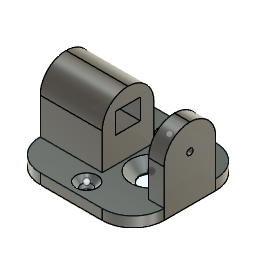
motorframe (Autodesk Fusion 360 design; units mm, degrees)
Autodesk Fusion 360 part; units mm, degrees
sketch "Skizze3" plane through (0, 0, 0) normal (0, 0, 1) x (1, 0, 0)
  line L0 (0, 0) -> (60, 0)
  line L1 (60, 0) -> (60, 55)
  line L2 (60, 55) -> (0, 55)
  line L3 (0, 55) -> (0, 0)
  line L4 (60, 55) -> (0, 55)
  line L5 (0, 55) -> (0, 0)
  line L6 (0, 0) -> (60, 0)
  line L7 (60, 0) -> (60, 55)
  line L8 (0, 15) -> (60, 15)
  line L9 (0, 40) -> (60, 40)
  line L10 (30, 40) -> (52.5, 40)
  line L11 (52.5, 40) -> (52.5, 15)
  line L12 (52.5, 15) -> (30, 15)
  line L13 (30, 15) -> (30, 40)
  point P0 (30, 7.5)
  point P1 (30, 47.5)
  dimension "d5" = 55
  dimension "d6" = 60
  dimension "d11" = 7.5
  dimension "d12" = 7.5
  dimension "d13" = 30
  dimension "d14" = 30
  dimension "d15" = 15
  dimension "d16" = 15
  dimension "d17" = 30
  dimension "d18" = 7.5
  dimension "d19" = 22.5
  constraint horizontal L0
  constraint vertical L1
  constraint horizontal L2
  constraint vertical L3
  constraint coincident L0.start L3.end
  constraint horizontal L4
  constraint vertical L5
  constraint horizontal L6
  constraint vertical L7
  constraint coincident L3 L8.start
  constraint coincident L7 L8.end
  constraint perpendicular L7 L8
  constraint coincident L5 L9.start
  constraint coincident L7 L9.end
  constraint perpendicular L7 L9
  constraint horizontal L10
  constraint vertical L11
  constraint horizontal L12
  constraint vertical L13
  constraint coincident L8 L11.end
  constraint coincident L9 L10.start
  measures "d5" distance of L0.start L2.end
  measures "d6" distance of L1.end L2.end
  measures "d11" distance of L4 P1
  measures "d12" distance of L0 P0
  measures "d13" distance of L5 P0
  measures "d14" distance of L3 P1
  measures "d15" distance of L0.end L8.end
  measures "d16" distance of L1.end L9.end
  measures "d17" distance of L3 L13
  measures "d18" distance of L1 L11
  measures "d19" distance of L11 L13
extrude "Extrusion2" add sketch "Skizze3" along normal blind 5
fillet "Abrundung2" radius 15 4 edges at (0, 55, 2.5) (0, 0, 2.5) (60, 0, 2.5) (60, 55, 2.5)
sketch "Skizze4" plane through (0, 0, 0) normal (0, 0, 1) x (1, 0, 0)
  line L0 (0, 15) -> (30, 15)
  line L1 (30, 15) -> (30, 40)
  line L2 (30, 40) -> (0, 40)
  line L3 (0, 40) -> (0, 15)
  point P0 (0, 15)
  point P1 (30, 40)
  constraint horizontal L0
  constraint vertical L1
  constraint horizontal L2
  constraint vertical L3
  constraint coincident P1 L1.end
  constraint coincident P0 L0.start
sketch "Skizze5" plane through (0, 0, 5) normal (0, 0, 1) x (-1, 0, 0)
  arc A0 (-60, -40) -> (-45, -55) centre (-45, -40) ccw
  line L0 (-45, -55) -> (-15, -55)
  arc A1 (-15, -55) -> (0, -40) centre (-15, -40) ccw
  line L1 (0, -40) -> (0, -15)
  arc A2 (0, -15) -> (-15, 0) centre (-15, -15) ccw
  line L2 (-15, 0) -> (-45, 0)
  arc A3 (-45, 0) -> (-60, -15) centre (-45, -15) ccw
  line L3 (-60, -15) -> (-60, -40)
  line L4 (-60, -15) -> (-52.5, -15)
  line L5 (-52.5, -15) -> (-52.5, -40)
  line L6 (-52.5, -40) -> (-60, -40)
  line L7 (-60, -40) -> (-60, -15)
  dimension "d20" = 7.5
  dimension "d21" = 25
  constraint horizontal L4
  constraint vertical L5
  constraint horizontal L6
  constraint vertical L7
  constraint coincident A3.end L3.start
  measures "d20" distance of L5 L7
  measures "d21" distance of L4 L6
extrude "Extrusion3" add sketch "Skizze5" along normal blind 30 contours L3 L4 L5 L6 L7
fillet "Abrundung3" radius 12.5 2 edges at (56.25, 15, 35) (56.25, 40, 35)
extrude "Extrusion4" add sketch "Skizze3" along normal blind 35 contours L3 L5 L8 L9 L13
fillet "Abrundung4" radius 12.5 2 edges at (15, 15, 35) (15, 40, 35)
sketch "Skizze6" plane through (0, 0, 5) normal (0, 0, 1) x (-1, 0, 0)
  line L0 (-30, -15) -> (0, -15)
  arc A0 (0, -15) -> (-15, 0) centre (-15, -15) ccw
  line L1 (-15, 0) -> (-45, 0)
  arc A1 (-45, 0) -> (-60, -15) centre (-45, -15) ccw
  line L2 (-60, -15) -> (-52.5, -15)
  line L3 (-52.5, -15) -> (-52.5, -40)
  line L4 (-52.5, -40) -> (-60, -40)
  arc A2 (-60, -40) -> (-45, -55) centre (-45, -40) ccw
  line L5 (-45, -55) -> (-15, -55)
  arc A3 (-15, -55) -> (0, -40) centre (-15, -40) ccw
  line L6 (0, -40) -> (-30, -40)
  line L7 (-30, -40) -> (-30, -15)
  point P0 (-30, -7.5)
  point P1 (-30, -47.5)
  point P2 (-41.25, -27.5)
  dimension "d48" = 27.5
  dimension "d49" = 27.5
  dimension "d50" = 11.25
  dimension "d51" = 11.25
  measures "d48" distance of L1 P2
  measures "d49" distance of L5 P2
  measures "d50" distance of L7 P2
  measures "d51" distance of L3 P2
hole "Bohrung1" at (30, 7.5, 5) at (30, 47.5, 5) direction (0, 0, -1) diameter 5.5 depth 33 tip angle 180 countersink diameter 10.4 countersink angle 90
sketch "Skizze7" plane through (60, 0, 0) normal (1, 0, 0) x (0, 1, 0)
  arc A0 (40, 22.5) -> (27.5, 35) centre (27.5, 22.5) ccw
  arc A1 (27.5, 35) -> (15, 22.5) centre (27.5, 22.5) ccw
  line L0 (15, 22.5) -> (15, 5)
  line L1 (15, 5) -> (15, 0)
  line L2 (15, 0) -> (40, 0)
  line L3 (40, 0) -> (40, 5)
  line L4 (40, 5) -> (40, 22.5)
  line L5 (0, 0) -> (55, 0)
  point P0 (27.5, 22.5)
  dimension "d35" = 12.5
  dimension "d36" = 22.5
  constraint coincident P0 A0.centre
  measures "d35" distance of A0.start P0
  measures "d36" distance of P0 L5
hole "Bohrung2" at (60, 27.5, 22.5) direction (-1, 0, 0) diameter 3 depth 33 tip angle 180
sketch "Skizze8" plane through (0, 0, 0) normal (-1, 0, 0) x (0, -1, 0)
  arc A0 (-27.5, 35) -> (-40, 22.5) centre (-27.5, 22.5) ccw
  line L0 (-40, 22.5) -> (-40, 5)
  line L1 (-40, 5) -> (-40, 0)
  line L2 (-40, 0) -> (-15, 0)
  line L3 (-15, 0) -> (-15, 5)
  line L4 (-15, 5) -> (-15, 22.5)
  arc A1 (-15, 22.5) -> (-27.5, 35) centre (-27.5, 22.5) ccw
  line L5 (-33.5, 27.5) -> (-21.5, 27.5)
  line L6 (-21.5, 27.5) -> (-21.5, 17.5)
  line L7 (-21.5, 17.5) -> (-33.5, 17.5)
  line L8 (-33.5, 17.5) -> (-33.5, 27.5)
  line L9 (-55, 0) -> (0, 0)
  dimension "d40" = 12
  dimension "d41" = 10
  dimension "d42" = 6.5
  dimension "d43" = 6.5
  dimension "d44" = 17.5
  dimension "d45" = 7.5
  constraint horizontal L5
  constraint vertical L6
  constraint horizontal L7
  constraint vertical L8
  measures "d40" distance of L5.start L5.end
  measures "d41" distance of L5 L7
  measures "d42" distance of L0 L8
  measures "d43" distance of L4 L6
  measures "d44" distance of L7 L9
  measures "d45" distance of A0.start L5
extrude "Extrusion5" cut sketch "Skizze8" against normal blind 30 contours L5 L6 L7 L8
sketch "Skizze9" plane through (0, 0, 0) normal (0, 0, 1) x (1, 0, 0)
  point P0 (42.3928, 28.246)
  point P1 (43.9941, 27.6171)
  constraint coincident P0
  constraint coincident P1
hole "Bohrung3" at (41.25, 27.5, 5) direction (0, 0, -1) diameter 11 depth 10 tip angle 180 countersink diameter 20 countersink angle 90
extrude "Extrusion1" [suppressed]
fillet "Abrundung1" [suppressed]
named bodies: "Seilwinde"
